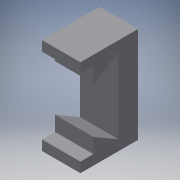
# Autodesk Inventor part: tester
Saved by Autodesk Inventor 2018 (Build 220112000, 112)
## iProperties
Created: 2018-09-13
Part Number: tester
Material: Generic
Document SubType Name: Modeling
Designer: David
Density: 1 g/cm^3
Appearance: Default
Author: David
Autodesk Inventor part; units mm, degrees
ref_plane "YZ Plane" through (0, 0, 0) normal (1, 0, 0) x (0, 1, 0)
ref_plane "XZ Plane" through (0, 0, 0) normal (0, 1, 0) x (-1, 0, 0)
ref_plane "XY Plane" through (0, 0, 0) normal (0, 0, 1) x (1, 0, 0)
sketch "Sketch1" plane through (0, 0, 0) normal (1, 0, 0) x (0, 1, 0)
  line L0 (-7.5, -12.5) -> (7.5, -12.5)
  line L1 (7.5, -12.5) -> (7.5, 12.5)
  line L2 (7.5, 12.5) -> (-7.5, 12.5)
  line L3 (-7.5, 12.5) -> (-7.5, -12.5)
  line L4 (-7.5, -12.5) -> (7.5, 12.5) construction
  line L5 (7.5, -12.5) -> (-7.5, 12.5) construction
  point P0 (0, 0)
  dimension "d0" = 25
  dimension "d1" = 15
  constraints: 12 end point, 2 midpoint, 2 parallel, 1 horizontal, 1 perpendicular
  measures "d0" distance of L0.end L1.end
  measures "d1" distance of L1.end L2.end
extrude "Extrusion1" add sketch "Sketch1" along normal blind 10
sketch "Sketch2" plane through (10, 0, 0) normal (1, 0, 0) x (0, 0, -1)
  line L0 (9.5, -4.5) -> (5.3472, -4.5) projected
  line L1 (9.5, -7.5) -> (9.5, -4.5) projected
  line L2 (9.5, -7.5) -> (22, -7.5) projected
  line L3 (22, 12.5) -> (22, -7.5) projected
  line L4 (-35, 12.5) -> (22, 12.5) projected
  line L5 (-35, 12.5) -> (-35, 59.5) projected
  line L6 (-45, 59.5) -> (-35, 59.5) projected
  line L7 (-45, 59.5) -> (-45, -7.5) projected
  line L8 (-45, -7.5) -> (-9.5, -7.5) projected
  line L9 (-9.5, -4.5) -> (-9.5, -7.5) projected
  line L10 (-5.3472, -4.5) -> (-9.5, -4.5) projected
  line L11 (-9.1, 2) -> (-5.3472, -4.5) projected
  line L12 (9.1, 2) -> (-9.1, 2) projected
  line L13 (5.3472, -4.5) -> (9.1, 2) projected
  line L14 (-9.5, -7.5) -> (9.5, -7.5)
  line L15 (-9.9, -7.1) -> (-44.6, -7.1)
  line L16 (-44.6, -7.1) -> (-44.6, 59.1)
  line L17 (-44.6, 59.1) -> (-35.4, 59.1)
  line L18 (-35.4, 59.1) -> (-35.4, 12.1)
  line L19 (-35.4, 12.1) -> (21.6, 12.1)
  line L20 (21.6, 12.1) -> (21.6, -7.1)
  line L21 (21.6, -7.1) -> (9.9, -7.1)
  line L22 (9.9, -7.1) -> (9.9, -4.1)
  line L23 (9.9, -4.1) -> (6.04, -4.1)
  line L24 (6.04, -4.1) -> (9.7928, 2.4)
  line L25 (9.7928, 2.4) -> (-9.7928, 2.4)
  line L26 (-9.7928, 2.4) -> (-6.04, -4.1)
  line L27 (-6.04, -4.1) -> (-9.9, -4.1)
  line L28 (-9.9, -4.1) -> (-9.9, -7.1)
  line L29 (-9.9, -7.1) -> (-9.9, -7.5)
  line L30 (-12.5, -7.5) -> (12.5, -7.5) projected
  line L31 (9.9, -7.1) -> (9.9, -7.5)
  line L32 (-12.5, -7.5) -> (12.5, -7.5) projected
  point P0 (0, 0)
  dimension "d4" = 0.4
  constraints: 34 end point, 3 perpendicular, 2 point on line, 13 other
  measures "d4" distance between parallel lines of L9 L28
extrude "Extrusion2" cut sketch "Sketch2" against normal blind 10 contours L1 L14 L9 L10 L11 L12 L13 L0 | L0 L13 L12 L11 L10 L9 L8 L29 L28 L27 L26 L25 L24 L23 L22 L31 L2 L1
body "Solid1"
